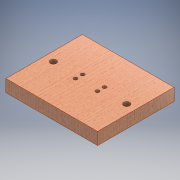
# Autodesk Inventor part: base de madera grande
Saved by Autodesk Inventor 2018 (Build 220112000, 112)
## iProperties
Created: 2019-05-20
Part Number: base de madera grande
Material: Generic
Document SubType Name: Modeling
Designer: Ivan
Density: 1 g/cm^3
Appearance: Default
Author: Ivan
Autodesk Inventor part; units mm, degrees
ref_plane "YZ Plane" through (0, 0, 0) normal (1, 0, 0) x (0, 1, 0)
ref_plane "XZ Plane" through (0, 0, 0) normal (0, 1, 0) x (-1, 0, 0)
ref_plane "XY Plane" through (0, 0, 0) normal (0, 0, 1) x (1, 0, 0)
sketch "Sketch1" plane through (0, 0, 0) normal (0, 0, 1) x (1, 0, 0)
  line L0 (-150, 125) -> (150, 125)
  line L1 (150, 125) -> (150, -125)
  line L2 (150, -125) -> (-150, -125)
  line L3 (-150, -125) -> (-150, 125)
  point P0 (0, 0)
  point P1 (0, 125)
  point P2 (150, 0)
  dimension "d0" = 300
  dimension "d1" = 250
  constraints: 8 end point, 2 midpoint, 2 parallel, 1 horizontal, 1 horizontal alignment, 1 perpendicular, 1 vertical alignment
  measures "d0" distance of L0.start L0.end
  measures "d1" distance of L0.end L1.end
extrude "Extrusion1" add sketch "Sketch1" along normal blind 40.35
sketch "Sketch2" plane through (0, 0, 40.35) normal (0, 0, 1) x (1, 0, 0)
  circle A0 centre (-120, 0) radius 5
  line L0 (150, 125) -> (-150, 125) construction
  line L1 (0, 125) -> (0, -125) construction
  line L2 (-150, -125) -> (150, -125) construction
  circle A1 centre (120, 0) radius 5
  point P0 (0, 0)
  dimension "d4" = 10
  dimension "d5" = 120
  constraints: 2 centre point, 2 end point, 2 midpoint, 1 horizontal alignment, 1 symmetric about line, 1 other
  measures "d4" diameter of A0
  measures "d5" distance of point (0, 0) A0.centre
hole "Hole1" at (-120, 0, 40.35) at (120, 0, 40.35) direction (0, 0, -1) diameter 10 end through all counterbore diameter 20 counterbore depth 15
sketch "Sketch4" plane through (0, 0, 40.35) normal (0, 0, 1) x (1, 0, 0)
  circle A0 centre (-36, 11.5) radius 2
  line L0 (150, 125) -> (-150, 125) construction
  line L1 (0, 125) -> (0, -125) construction
  line L2 (-150, -125) -> (150, -125) construction
  line L3 (150, -125) -> (150, 125) construction
  line L4 (150, 0) -> (-150, 0) construction
  line L5 (-150, 125) -> (-150, -125) construction
  circle A1 centre (-36, -11.5) radius 2
  line L6 (0, -125) -> (0, 125) construction
  circle A2 centre (36, 11.5) radius 2
  circle A3 centre (36, -11.5) radius 2
  point P0 (0, 0)
  dimension "d13" = 4
  dimension "d14" = 11.5
  dimension "d15" = 36
  constraints: 6 end point, 5 symmetric about line, 4 centre point, 4 midpoint, 3 other
  measures "d13" diameter of A0
  measures "d14" vertical distance of point (0, 0) A0.centre
  measures "d15" horizontal distance of point (0, 0) A0.centre
hole "Hole2" at (-36, 11.5, 40.35) at (36, 11.5, 40.35) at (36, -11.5, 40.35) at (-36, -11.5, 40.35) direction (0, 0, -1) diameter 4 end through all counterbore diameter 12 counterbore depth 10
body "Solid1"
